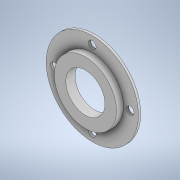
# Autodesk Inventor part: tensorpolea
Saved by Autodesk Inventor 2021 (Build 250183000, 183)
## iProperties
Created: 2021-01-03
Part Number: tensorpolea
Material: Generic
Document SubType Name: Modeling
Designer: Cristobal
Density: 1 g/cm^3
Appearance: Default
Author: Cristobal
Autodesk Inventor part; units mm, degrees
ref_plane "YZ Plane" through (0, 0, 0) normal (1, 0, 0) x (0, 1, 0)
ref_plane "XZ Plane" through (0, 0, 0) normal (0, 1, 0) x (-1, 0, 0)
ref_plane "XY Plane" through (0, 0, 0) normal (0, 0, 1) x (1, 0, 0)
sketch "Sketch1" plane through (0, 0, 0) normal (0, 0, 1) x (1, 0, 0)
  circle A0 centre (0, 0) radius 40
  circle A1 centre (0, 0) radius 27
  circle A2 centre (0, 0) radius 17
  circle A3 centre (0, 33) radius 3.3
  circle A4 centre (-33, 0) radius 3.3
  circle A5 centre (0, -33) radius 3.3
  circle A6 centre (33, 0) radius 3.3
  dimension "d0" = 80
  dimension "d1" = 54
  dimension "d2" = 34
  dimension "d4" = 6.6
  dimension "d5" = 6.6
  dimension "d6" = 6.6
  dimension "d7" = 6.6
  constraints: 7 centre point, 3 coincident
  measures "d0" diameter of A0
  measures "d1" diameter of A1
  measures "d2" diameter of A2
  measures "d4" diameter of A3
  measures "d5" diameter of A4
  measures "d6" diameter of A5
  measures "d7" diameter of A6
extrude "Extrusion1" add sketch "Sketch1" along normal blind 2 contours A0
extrude "Extrusion2" add sketch "Sketch1" along normal blind 8 contours A1
body "Solid1"
